Autodesk Fusion 360 part; units mm, degrees
note: some values were not read from the file. Set by a fixed rule: the direction of a hole.
(part 3 of 4)
sketch "草图3" plane through (0, 0, 0) normal (0, 0, 1) x (-1, 0, 0)
  circle A0 centre (-13.5, -30) radius 1.6
  circle A1 centre (0, -30) radius 9
  circle A2 centre (13.5, -30) radius 1.6
  circle A3 centre (6.75, -41.6913) radius 1.6
  circle A4 centre (6.75, -18.3087) radius 1.6
  circle A5 centre (-6.75, -18.3087) radius 1.6
  circle A6 centre (-6.75, -41.6913) radius 1.6
  arc A7 (27.4762, -17.824) -> (28.5, -13.9083) centre (20.5, -13.9083) ccw
  line L0 (28.5, -13.9083) -> (28.5, 0)
  line L1 (28.5, 0) -> (-28.5, 0)
  line L2 (-28.5, 0) -> (-28.5, -13.9083)
  arc A8 (-28.5, -13.9083) -> (-27.4762, -17.824) centre (-20.5, -13.9083) ccw
  line L3 (-27.4762, -17.824) -> (-15.6964, -38.8105)
  arc A9 (-15.6964, -38.8105) -> (15.6964, -38.8105) centre (0, -30) ccw
  line L4 (15.6964, -38.8105) -> (27.4762, -17.824)
  line L5 (0, 0) -> (0, -30) construction
  line L6 (-23.5, -6) -> (-23.5, -14.6927)
  line L7 (-23.5, -14.6927) -> (-18.1186, -24.28)
  line L8 (-23.5, -6) -> (-3, -6)
  line L9 (-3, -6) -> (-3, -11.2383)
  arc A10 (-3, -11.2383) -> (-18.1186, -24.28) centre (0, -30) ccw
  line L10 (-23.5, -6) -> (-28.5, -6) construction
  line L11 (-23.5, -6) -> (-23.5, 0) construction
  line L12 (-18.1186, -24.28) -> (-22.4787, -26.7274) construction
  line L13 (-3, -6) -> (0, -6) construction
  line L14 (23.5, -6) -> (23.5, -14.6927)
  line L15 (23.5, -6) -> (3, -6)
  line L16 (3, -6) -> (3, -11.2383)
  arc A11 (18.1186, -24.28) -> (3, -11.2383) centre (0, -30) ccw
  line L17 (23.5, -14.6927) -> (18.1186, -24.28)
  dimension "d21" = 5
  dimension "d22" = 19
  dimension "d23" = 3
  dimension "d26" = 6
  constraint coincident L5.start origin
  constraint coincident A1.centre A9.centre
  constraint vertical L6
  constraint perpendicular L6 L8
  constraint perpendicular L8 L9
  constraint parallel L3 L7
  constraint coincident L2 L10.end
  constraint perpendicular L2 L10
  constraint coincident L1 L11.end
  constraint perpendicular L1 L11
  constraint coincident L3 L12.end
  constraint perpendicular L3 L12
  constraint coincident L5 L13.end
  constraint perpendicular L5 L13
  constraint symmetric L5 L6.start L14.start
  constraint symmetric L5 L6.end L14.end
  constraint symmetric L5 L8.end L15.end
  constraint symmetric L5 L9.end L16.end
  constraint symmetric L5 L7.end A11.start
  constraint symmetric L5 A10 A11
  constraint equal L10 L12
  measures "d21" distance of L6.start L10.end
  measures "d22" radius of A10
  measures "d23" distance of L8.end L13.end
  measures "d26" distance of L6.start L11.end
extrude "拉伸4" cut sketch "草图3" against normal blind 8 contours L6 L7 L8 L9 A10 | L14 L15 L16 A11 L17
fillet "圆角2" radius 2 8 edges at (18.1186, 24.28, -4) (-18.1186, 24.28, -4) (23.5, 6, -4) (3, 6, -4) (-23.5, 6, -4) (-3, 6, -4) (-3, 11.2383, -4) (3, 11.2383, -4)
fillet "圆角2" radius 6 2 edges at (-23.5, 14.6927, -4) (23.5, 14.6927, -4)
sketch "草图4" plane through (0, 0, 0) normal (0, 0, 1) x (-1, 0, 0)
  arc A0 (27.4762, -17.824) -> (28.5, -13.9083) centre (20.5, -13.9083) ccw
  line L0 (28.5, -13.9083) -> (28.5, 0)
  line L1 (28.5, 0) -> (-28.5, 0)
  line L2 (-28.5, 0) -> (-28.5, -13.9083)
  arc A1 (-28.5, -13.9083) -> (-27.4762, -17.824) centre (-20.5, -13.9083) ccw
  line L3 (-27.4762, -17.824) -> (-15.6964, -38.8105)
  arc A2 (-15.6964, -38.8105) -> (15.6964, -38.8105) centre (0, -30) ccw
  line L4 (15.6964, -38.8105) -> (27.4762, -17.824)
  circle A3 centre (-6.75, -41.6913) radius 1.6
  circle A4 centre (-6.75, -18.3087) radius 1.6
  circle A5 centre (6.75, -18.3087) radius 1.6
  circle A6 centre (6.75, -41.6913) radius 1.6
  circle A7 centre (13.5, -30) radius 1.6
  circle A8 centre (0, -30) radius 9
  circle A9 centre (-13.5, -30) radius 1.6
  line L5 (-20.0922, -20.7639) -> (-22.7321, -16.0607)
  arc A10 (-23.5, -13.1239) -> (-22.7321, -16.0607) centre (-17.5, -13.1239) ccw
  line L6 (-23.5, -13.1239) -> (-23.5, -8)
  arc A11 (-21.5, -6) -> (-23.5, -8) centre (-21.5, -8) ccw
  line L7 (-21.5, -6) -> (-5, -6)
  arc A12 (-3, -8) -> (-5, -6) centre (-5, -8) ccw
  line L8 (-3, -8) -> (-3, -9.6039)
  arc A13 (-4.5238, -11.5464) -> (-3, -9.6039) centre (-5, -9.6039) ccw
  arc A14 (-4.5238, -11.5464) -> (-16.6007, -20.7579) centre (0, -30) ccw
  arc A15 (-20.0922, -20.7639) -> (-16.6007, -20.7579) centre (-18.3481, -19.785) ccw
  line L9 (3, -9.6039) -> (3, -8)
  arc A16 (5, -6) -> (3, -8) centre (5, -8) ccw
  line L10 (5, -6) -> (21.5, -6)
  arc A17 (23.5, -8) -> (21.5, -6) centre (21.5, -8) ccw
  line L11 (23.5, -8) -> (23.5, -13.1239)
  arc A18 (22.7321, -16.0607) -> (23.5, -13.1239) centre (17.5, -13.1239) ccw
  line L12 (22.7321, -16.0607) -> (20.0922, -20.7639)
  arc A19 (16.6007, -20.7579) -> (20.0922, -20.7639) centre (18.3481, -19.785) ccw
  arc A20 (16.6007, -20.7579) -> (4.5238, -11.5464) centre (0, -30) ccw
  arc A21 (3, -9.6039) -> (4.5238, -11.5464) centre (5, -9.6039) ccw
  circle A22 centre (-13.5, -30) radius 3
  circle A23 centre (-6.75, -41.6913) radius 3
  circle A24 centre (6.75, -41.6913) radius 3
  circle A25 centre (13.5, -30) radius 3
  circle A26 centre (6.75, -18.3087) radius 3
  circle A27 centre (-6.75, -18.3087) radius 3
  dimension "d31" = 6
  dimension "d33" = 360
  constraint concentric A9 A22
  measures "d31" diameter of A22
extrude "拉伸5" cut sketch "草图4" against normal blind 3.2 contours A22 | A23 | A24 | A25 | A26 | A27

design "深沟球20，27，4"
part number: 2026-07-22-11-56-50-553
Autodesk Fusion 360 part; units mm, degrees
sketch "草图1" plane through (0, 0, 0) normal (0, 0, 1) x (1, 0, 0)
  circle A0 centre (0, 0) radius 13.5
  circle A1 centre (0, 0) radius 10
  dimension "d1" = 27
  dimension "d2" = 20
  constraint coincident A0.centre A1.centre
  constraint concentric A0 A1
  measures "d1" diameter of A0
  measures "d2" diameter of A1
extrude "拉伸1" add sketch "草图1" along normal blind 3.2
sketch "草图2" plane through (0, 0, 3.2) normal (0, 0, 1) x (1, 0, 0)
  circle A0 centre (0, 0) radius 10
  circle A1 centre (0, 0) radius 13.5
  circle A2 centre (0, 0) radius 14.25
  dimension "d5" = 28.5
  constraint coincident A0.centre A1.centre
  measures "d5" diameter of A2
extrude "拉伸2" add sketch "草图2" along normal blind 0.8 contours A1 | A2

design "yaw输出cnc"
part number: 2026-07-21-18-54-59-892
Autodesk Fusion 360 part; units mm, degrees
sketch "草图1" plane through (0, 0, 0) normal (0, 0, 1) x (1, 0, 0)
  circle A0 centre (0, 0) radius 17.5
  circle A1 centre (0, 0) radius 13.5 construction
  circle A2 centre (-13.5, 0) radius 1.8
  circle A3 centre (-6.75, -11.6913) radius 1.8
  circle A4 centre (6.75, -11.6913) radius 1.8
  circle A5 centre (13.5, 0) radius 1.8
  circle A6 centre (6.75, 11.6913) radius 1.8
  circle A7 centre (-6.75, 11.6913) radius 1.8
  dimension "d1" = 35
  dimension "d2" = 27
  dimension "d3" = 3.6
  dimension "d5" = 360
  constraint coincident A0.centre A1.centre
  constraint concentric A0 A1
  constraint coincident A1 A2.centre
  constraint horizontal A2.centre A5.centre
  measures "d1" diameter of A0
  measures "d2" diameter of A1
  measures "d3" diameter of A2
extrude "拉伸1" add sketch "草图1" along normal blind 7.6
sketch "草图2" plane through (0, 0, 7.6) normal (0, 0, 1) x (-1, 0, 0)
  circle A0 centre (-6.75, 11.6913) radius 1.8
  circle A1 centre (6.75, -11.6913) radius 1.8
  circle A2 centre (13.5, 0) radius 1.8
  circle A3 centre (-13.5, 0) radius 1.8
  circle A4 centre (-6.75, -11.6913) radius 1.8
  circle A5 centre (6.75, 11.6913) radius 1.8
  circle A6 centre (0, 0) radius 17.5
  circle A7 centre (0, 0) radius 19
  dimension "d9" = 38
  constraint concentric A6 A7
  measures "d9" diameter of A7
extrude "拉伸2" add sketch "草图2" along normal blind 6 contours A6 | A7
sketch "草图10" plane through (0, 0, 13.6) normal (0, 0, 1) x (-1, 0, 0)
  circle A0 centre (-6.75, -11.6913) radius 1.8
  circle A1 centre (6.75, -11.6913) radius 1.8
  circle A2 centre (13.5, 0) radius 1.8
  circle A3 centre (-13.5, 0) radius 1.8
  circle A4 centre (-6.75, 11.6913) radius 1.8
  circle A5 centre (6.75, 11.6913) radius 1.8
  circle A6 centre (0, 0) radius 19
  circle A7 centre (0, 0) radius 8
  dimension "d51" = 16
  constraint coincident A6.centre A7.centre
  measures "d51" diameter of A7
extrude "拉伸9" cut sketch "草图10" against normal blind 47 contours A7
sketch "草图11" plane through (0, 0, 13.6) normal (0, 0, 1) x (-1, 0, 0)
  circle A0 centre (0, 0) radius 8
  circle A1 centre (-6.75, -11.6913) radius 1.8
  circle A2 centre (6.75, -11.6913) radius 1.8
  circle A3 centre (13.5, 0) radius 1.8
  circle A4 centre (-13.5, 0) radius 1.8
  circle A5 centre (-6.75, 11.6913) radius 1.8
  circle A6 centre (6.75, 11.6913) radius 1.8
  circle A7 centre (0, 0) radius 19
  line L0 (0, 0) -> (24.6202, -4.3412)
  line L1 (0, 0) -> (24, 0)
  line L2 (0, 0) -> (24.6202, 4.3412)
  circle A8 centre (0, 0) radius 25
  circle A9 centre (0, 0) radius 19
  dimension "d56" = 10
  dimension "d57" = 10
  dimension "d63" = 50
  constraint coincident A0.centre A7.centre
  constraint horizontal L1
  constraint concentric A0 A8
  constraint coincident L0.end A8
  constraint coincident L2.end A8
  measures "d56" angle of L0 L1
  measures "d57" angle of L1 L2
  measures "d63" diameter of A8
extrude "拉伸10" add sketch "草图11" against normal blind 3 contours A7 L0 L2 A8 A9 picked at (22.8867, -2.1872)
fillet "圆角1" radius 1 4 edges at (-18.7113, 3.2993, 12.1) (-24.6202, 4.3412, 12.1) (-24.6202, -4.3412, 12.1) (-18.7113, -3.2993, 12.1)
equation "d38 = ( 45 / 4 ) * 1 mm"
equation "d69 = '7.4'"

design "l2电机固定前"
part number: 2026-07-22-11-09-26-482
Autodesk Fusion 360 part; units mm, degrees
sketch "草图1" plane through (0, 0, 0) normal (0, 0, 1) x (1, 0, 0)
  circle A0 centre (0, 50.1368) radius 25 construction
  circle A1 centre (0, 50.1368) radius 20
  circle A2 centre (0, 50.1368) radius 30
  circle A3 centre (-22.6577, 60.7023) radius 1.6
  circle A4 centre (-20.4788, 35.7974) radius 1.6
  circle A5 centre (2.1789, 25.232) radius 1.6
  circle A6 centre (22.6577, 39.5714) radius 1.6
  circle A7 centre (20.4788, 64.4762) radius 1.6
  circle A8 centre (-2.1789, 75.0417) radius 1.6
  line L0 (-22.5, 10.1368) -> (22.5, 10.1368)
  line L1 (0, 10.1368) -> (0, 50.1368)
  line L2 (6.1726, 76.5877) -> (6.1726, 78.4678)
  circle A9 centre (0, 50.1368) radius 18
  line L3 (0, 50.1368) -> (0, 87.9264)
  line L4 (-29.4017, 44.1753) -> (-22.5, 10.1368)
  line L5 (22.5, 10.1368) -> (29.4017, 44.1753)
  line L6 (-22.6577, 60.7023) -> (0, 50.1368) construction
  dimension "d1" = 50
  dimension "d2" = 40
  dimension "d3" = 60
  dimension "d4" = 3.2
  dimension "d6" = 360
  dimension "d9" = 40
  dimension "d12" = 22.5
  dimension "d79" = 65
  constraint concentric A0 A1
  constraint concentric A1 A2
  constraint horizontal L0
  constraint vertical origin A0.centre
  constraint midpoint L0 L1.start
  constraint coincident A0.centre A1.centre
  constraint coincident A0 A3.centre
  constraint parallel L2 L3
  constraint vertical L1
  constraint coincident A2 L4.start
  constraint coincident A2 L5.end
  constraint tangent A2 L5
  constraint tangent A2 L4
  constraint coincident A3.centre L6.start
  constraint vertical L3
  measures "d1" diameter of A0
  measures "d2" diameter of A1
  measures "d3" diameter of A2
  measures "d4" diameter of A3
  measures "d9" distance of A0.centre L0
  measures "d12" distance of L0.start L1
  measures "d79" angle of L3 L6
extrude "拉伸1" add sketch "草图1" along normal blind 4 contours A1 A2 L1 L3 | A1 A2 L1 L3 | A2 L0 L1 L4 | A2 L0 L1 L5 | A3 | A4 | A5 | A6 | A7 | A8
sketch "草图2" plane through (0, 0, 0) normal (0, 0, -1) x (-1, 0, 0)
  circle A0 centre (-17.5, 13.1368) radius 1.65
  circle A1 centre (0, 13.1368) radius 1.65
  circle A2 centre (17.5, 13.1368) radius 1.65
  line L0 (-29.4017, 44.1753) -> (-22.5, 10.1368)
  line L1 (-22.5, 10.1368) -> (22.5, 10.1368)
  line L2 (22.5, 10.1368) -> (29.4017, 44.1753)
  arc A3 (29.4017, 44.1753) -> (-29.4017, 44.1753) centre (0, 50.1368) ccw
  circle A4 centre (0, 50.1368) radius 20
  dimension "d13" = 3.3
  dimension "d18" = 35
  dimension "d19" = 0
  dimension "d29" = 3
  dimension "d40" = 5
  measures "d13" diameter of A0
  measures "d29" distance of A0.centre L1
  measures "d40" horizontal distance of A0.centre L0.end
extrude "拉伸2" cut sketch "草图2" against normal blind 10 contours A0 | A1 | A2
sketch "草图4" plane through (0, 0, 0) normal (0, 0, -1) x (-1, 0, 0)
  line L0 (-29.4017, 44.1753) -> (-22.5, 10.1368)
  line L1 (-22.5, 10.1368) -> (22.5, 10.1368)
  line L2 (22.5, 10.1368) -> (29.4017, 44.1753)
  arc A0 (29.4017, 44.1753) -> (-29.4017, 44.1753) centre (0, 50.1368) ccw
  circle A1 centre (-17.5, 13.1368) radius 1.65
  circle A2 centre (17.5, 13.1368) radius 1.65
  circle A3 centre (0, 13.1368) radius 1.65
  circle A4 centre (-17.5, 13.1368) radius 3
  line L3 (-20.5, 13.1368) -> (-20.5, 10.1368)
  line L4 (-14.5, 13.1368) -> (-14.5, 10.1368)
  circle A5 centre (0, 13.1368) radius 3
  line L5 (3, 13.1368) -> (3, 10.1368)
  line L6 (-3, 13.1368) -> (-3, 10.1368)
  circle A6 centre (17.5, 13.1368) radius 3
  line L7 (20.5, 13.1368) -> (20.5, 10.1368)
  line L8 (14.5, 13.1368) -> (14.5, 10.1368)
  circle A7 centre (0, 50.1368) radius 20
  dimension "d36" = 35
  dimension "d37" = 0
  constraint concentric A1 A4
  constraint tangent L1 A4
  constraint coincident A4 L3.start
  constraint coincident L1 L3.end
  constraint tangent A4 L3
  constraint vertical L3
  constraint coincident A4 L4.start
  constraint coincident L1 L4.end
  constraint perpendicular L1 L4
  constraint tangent A4 L4
hole "孔1" at (2.1789, 25.232, 0) at (-20.4788, 35.7974, 0) at (-22.6577, 60.7023, 0) at (-2.1789, 75.0417, 0) at (20.4788, 64.4762, 0) at (22.6577, 39.5714, 0) direction (0, 0, 1) diameter 3.3 depth 7 tip angle 180 countersink diameter 6.3 countersink angle 90
sketch "草图5" plane through (0, 0, 0) normal (0, 0, 1) x (1, 0, 0)
  circle A0 centre (17.5, 13.1368) radius 1.65
  circle A1 centre (0, 13.1368) radius 1.65
  circle A2 centre (-17.5, 13.1368) radius 1.65
  circle A3 centre (0, 50.1368) radius 20
  line L0 (22.5, 10.1368) -> (29.4017, 44.1753)
  arc A4 (29.4017, 44.1753) -> (-29.4017, 44.1753) centre (0, 50.1368) ccw
  line L1 (-29.4017, 44.1753) -> (-22.5, 10.1368)
  line L2 (-22.5, 10.1368) -> (22.5, 10.1368)
  circle A5 centre (-25, 50.1368) radius 1.6
  circle A6 centre (12.5, 28.4862) radius 1.6
  circle A7 centre (12.5, 71.7875) radius 1.6
  circle A8 centre (-12.5, 71.7875) radius 1.6
  circle A9 centre (25, 50.1368) radius 1.6
  circle A10 centre (-12.5, 28.4862) radius 1.6
  circle A11 centre (0, 50.1368) radius 25
  line L3 (75, 70.1368) -> (-75, 70.1368)
  arc A12 (-75, 70.1368) -> (-75, 30.1368) centre (-75, 50.1368) ccw
  line L4 (-75, 30.1368) -> (75, 30.1368)
  arc A13 (75, 30.1368) -> (75, 70.1368) centre (75, 50.1368) ccw
  line L5 (75, 50.1368) -> (-75, 50.1368) construction
  line L6 (-40, 30.1368) -> (-3.2298, 25.3463)
  circle A14 centre (17.5, 13.1368) radius 1.65
  circle A15 centre (0, 13.1368) radius 1.65
  circle A16 centre (-17.5, 13.1368) radius 1.65
  circle A17 centre (0, 50.1368) radius 20
  line L7 (29.4017, 44.1753) -> (22.5, 10.1368)
  line L8 (22.5, 10.1368) -> (-22.5, 10.1368)
  line L9 (-22.5, 10.1368) -> (-29.4017, 44.1753)
  arc A18 (29.4017, 44.1753) -> (-29.4017, 44.1753) centre (0, 50.1368) ccw
  circle A19 centre (2.1789, 25.232) radius 3.15
  circle A20 centre (0, 50.1368) radius 30
  line L10 (3.2298, 25.3463) -> (40, 30.1368)
  circle A21 centre (22.6577, 39.5714) radius 3.15
  circle A22 centre (-2.1789, 75.0417) radius 3.15
  circle A23 centre (-20.4788, 35.7974) radius 3.15
  circle A24 centre (-22.6577, 60.7023) radius 3.15
  circle A25 centre (20.4788, 64.4762) radius 3.15
  line L11 (24.0557, 17.8092) -> (-24.0557, 17.8092)
  line L12 (24.0557, 17.8092) -> (-6.4705, 25.9887)
  point P0 (0, 50.1368)
  dimension "d46" = 50
  dimension "d47" = 20
  dimension "d48" = 40
  dimension "d75" = 60
  dimension "d76" = 40
  dimension "d84" = 15
  constraint concentric A3 A11
  constraint tangent L3 A12
  constraint tangent A12 L4
  constraint parallel L3 L4
  constraint tangent L4 A13
  constraint tangent L3 A13
  constraint horizontal L5
  constraint coincident P0 A3.centre
  constraint midpoint L5 P0
  constraint coincident L4 L6.start
  constraint coincident A11 L6.end
  constraint tangent A11 L6
  constraint concentric A17 A20
  constraint coincident A11 L10.start
  constraint coincident L4 L10.end
  constraint tangent A11 L10
  constraint coincident L7 L11.start
  constraint coincident L9 L11.end
  constraint horizontal L11
  constraint coincident A11 L12.end
  constraint tangent A11 L12
  measures "d46" diameter of A11
  measures "d47" radius of A12
  measures "d48" horizontal distance of P0 L6.start
  measures "d75" diameter of A20
  measures "d76" horizontal distance of P0 L10.end
  measures "d84" angle of L11 L12
extrude "拉伸5" add sketch "草图5" against normal blind 6 contours L1 L6 L9 A20 L11 L12 | L0 L1 L2 L7 L8 L9 L11
fillet "圆角1" radius 2 7 edges at (-22.5, 10.1368, -1) (22.5, 10.1368, 2) (22.5, 10.1368, -3) (24.0557, 17.8092, -3) (9.5476, 21.6966, -3) (-19.6739, 27.4887, -3) (-26.1904, 28.3377, -3)
sketch "草图6" plane through (0, 0, -6) normal (0, 0, -1) x (1, 0, 0)
  line L0 (-22.8249, -11.7394) -> (-25.6344, -25.5955)
  line L1 (20.8648, -10.1368) -> (-20.8648, -10.1368)
  line L2 (23.682, -15.9666) -> (22.8249, -11.7394)
  line L3 (0, 0) -> (0, -50.1368)
  line L4 (-21.7001, -21.2885) -> (-5, -17.1368)
  line L5 (-5, -17.1368) -> (-19.3031, -17.1368)
  line L6 (-19.3031, -17.1368) -> (-21.7001, -21.2885)
  line L7 (5, -17.1368) -> (19.3031, -17.1368)
  line L8 (19.3031, -17.1368) -> (21.7001, -21.2885)
  line L9 (21.7001, -21.2885) -> (5, -17.1368)
  arc A0 (9.0021, -21.5193) -> (-19.2373, -27.1167) centre (0, -50.1368) ccw
  circle A1 centre (17.5, -13.1368) radius 1.65
  circle A2 centre (0, -13.1368) radius 1.65
  circle A3 centre (-17.5, -13.1368) radius 1.65
  arc A4 (22.8249, -11.7394) -> (20.8648, -10.1368) centre (20.8648, -12.1368) ccw
  arc A5 (-20.8648, -10.1368) -> (-22.8249, -11.7394) centre (-20.8648, -12.1368) ccw
  line L10 (-23.4159, -27.9762) -> (-20.2614, -27.5652)
  line L11 (10.1198, -21.5433) -> (22.2396, -18.2958)
  arc A6 (-25.6344, -25.5955) -> (-23.4159, -27.9762) centre (-23.6743, -25.993) ccw
  arc A7 (-20.2614, -27.5652) -> (-19.2373, -27.1167) centre (-20.5198, -25.582) ccw
  arc A8 (9.0021, -21.5193) -> (10.1198, -21.5433) centre (9.6022, -19.6115) ccw
  arc A9 (22.2396, -18.2958) -> (23.682, -15.9666) centre (21.7219, -16.364) ccw
  dimension "d69" = 5
  dimension "d71" = 120
  constraint coincident L3.start origin
  constraint horizontal L5
  constraint symmetric L3 L4.start L8.end
  constraint symmetric L3 L4.end L7.start
  constraint symmetric L3 L5.end L7.end
  measures "d69" distance of L3 L4.end
  measures "d71" angle of L5 L6
sketch "草图7" plane through (0, 0, -6) normal (0, 0, -1) x (1, 0, 0)
  line L0 (-22.8249, -11.7394) -> (-25.6344, -25.5955)
  line L1 (23.682, -15.9666) -> (22.8249, -11.7394)
  circle A0 centre (-17.5, -13.1368) radius 3
  line L2 (-20.5, -13.1368) -> (-20.5, -10.1368)
  line L3 (-14.5, -13.1368) -> (-14.5, -10.0707)
  line L4 (20.8648, -10.1368) -> (-20.8648, -10.1368)
  arc A1 (9.0021, -21.5193) -> (-19.2373, -27.1167) centre (0, -50.1368) ccw
  circle A2 centre (17.5, -13.1368) radius 1.65
  circle A3 centre (0, -13.1368) radius 1.65
  circle A4 centre (-17.5, -13.1368) radius 1.65
  arc A5 (22.8249, -11.7394) -> (20.8648, -10.1368) centre (20.8648, -12.1368) ccw
  arc A6 (-20.8648, -10.1368) -> (-22.8249, -11.7394) centre (-20.8648, -12.1368) ccw
  line L5 (-23.4159, -27.9762) -> (-20.2614, -27.5652)
  line L6 (10.1198, -21.5433) -> (22.2396, -18.2958)
  arc A7 (-25.6344, -25.5955) -> (-23.4159, -27.9762) centre (-23.6743, -25.993) ccw
  arc A8 (-20.2614, -27.5652) -> (-19.2373, -27.1167) centre (-20.5198, -25.582) ccw
  arc A9 (9.0021, -21.5193) -> (10.1198, -21.5433) centre (9.6022, -19.6115) ccw
  arc A10 (22.2396, -18.2958) -> (23.682, -15.9666) centre (21.7219, -16.364) ccw
  dimension "d62" = 6
  constraint coincident A0 L2.start
  constraint coincident A0 L3.start
  constraint vertical L3
  constraint vertical L2
  constraint tangent A0 L3
  constraint tangent A0 L2
  constraint coincident L2.end L4
  measures "d62" diameter of A0
extrude "拉伸7" cut sketch "草图7" against normal blind 3 contours A0 L2 L4 | A0 | A0 L3 L4 | A4
pattern_linear "R-阵列2" count 3 spacing 17.5 along (1, 0, 0) of "拉伸7"

design "M3铝柱 55mm"
part number: 2026-08-11-12-14-30-494
Autodesk Fusion 360 part; units mm, degrees
sketch "草图1" plane through (0, 0, 0) normal (0, 1, 0) x (1, 0, 0)
  circle A0 centre (0, 0) radius 1.5
  circle A1 centre (0, 0) radius 3
  dimension "d1" = 3
  dimension "d2" = 6
  constraint coincident A0.centre A1.centre
  measures "d1" diameter of A0
  measures "d2" diameter of A1
extrude "拉伸1" add sketch "草图1" along normal mid plane 55 makes body 1
pattern_linear "R-阵列1" count 2 spacing 50 along (1, 0, 0) count 2 spacing 30 along (0, 0, 1) of bodies 1 makes body 2 at (52.9851, 9.1667, 0.2987) makes body 3 at (2.9851, 9.1667, 30.2987) makes body 4 at (52.9851, 9.1667, 30.2987)

design "深沟球35*44*5"
part number: 2026-07-21-18-41-33-064
Autodesk Fusion 360 part; units mm, degrees
sketch "草图1" plane through (0, 0, 0) normal (0, 0, 1) x (1, 0, 0)
  circle A0 centre (0, 0) radius 17.5
  circle A1 centre (0, 0) radius 22
  dimension "d1" = 35
  dimension "d2" = 44
  constraint coincident A0.centre A1.centre
  measures "d1" diameter of A0
  measures "d2" diameter of A1
extrude "拉伸1" add sketch "草图1" along normal blind 5

design "滑块底座"
part number: 2026-07-22-10-29-59-170
Autodesk Fusion 360 part; units mm, degrees
sketch "草图1" plane through (0, 0, 0) normal (0, 1, 0) x (1, 0, 0)
  line L0 (0, 0) -> (0, -4.5) construction
  line L1 (0, 0) -> (-20, 0)
  line L2 (-20, 0) -> (-20, -7)
  line L3 (-20, -7) -> (-8.6, -7)
  line L4 (-8.6, -7) -> (-8.6, -4.5)
  line L5 (-8.6, -4.5) -> (0, -4.5)
  line L6 (20, 0) -> (20, -7)
  line L7 (20, -7) -> (8.6, -7)
  line L8 (8.6, -7) -> (8.6, -4.5)
  line L9 (8.6, -4.5) -> (0, -4.5)
  line L10 (0, 0) -> (20, 0)
  dimension "d1" = 40
  dimension "d2" = 7
  dimension "d4" = 2.5
  dimension "d16" = 17.2
  constraint coincident L0.start L1.start
  constraint vertical L0
  constraint perpendicular L0 L1
  constraint perpendicular L1 L2
  constraint perpendicular L2 L3
  constraint perpendicular L3 L4
  constraint perpendicular L0 L5
  constraint symmetric L1.start L0 L10.start
  constraint symmetric L5.end L0 L9.end
  constraint symmetric L0 L3.end L7.end
  constraint symmetric L0 L4.end L8.end
  constraint symmetric L0 L2.end L6.end
  constraint horizontal L10
  measures "d1" distance of L2 L6
  measures "d2" distance of L1.end L2.end
  measures "d4" distance of L3.end L4.end
  measures "d16" distance of L4 L8
extrude "拉伸1" add sketch "草图1" along normal mid plane 22.5
sketch "草图2" plane through (0, 0, 0) normal (0, 0, 1) x (-1, 0, 0)
  line L0 (-8.6, 11.25) -> (-8.6, -11.25)
  line L1 (-8.6, -11.25) -> (8.6, -11.25)
  line L2 (8.6, -11.25) -> (8.6, 11.25)
  line L3 (8.6, 11.25) -> (-8.6, 11.25)
  line L4 (0, -11.25) -> (0, 11.25) construction
  line L5 (8.6, 0) -> (-8.6, 0) construction
  circle A0 centre (6, -4) radius 1.75
  circle A1 centre (-6, -4) radius 1.75
  circle A2 centre (6, 4) radius 1.75
  circle A3 centre (-6, 4) radius 1.75
  line L6 (20, 11.25) -> (20, -11.25)
  line L7 (20, -11.25) -> (-20, -11.25)
  line L8 (-20, -11.25) -> (-20, 11.25)
  line L9 (-20, 11.25) -> (20, 11.25)
  dimension "d7" = 3.5
  dimension "d8" = 8
  dimension "d9" = 12
  constraint midpoint L1 L4.start
  constraint perpendicular L1 L4
  constraint midpoint L2 L5.start
  constraint midpoint L0 L5.end
  constraint equal A0 A1
  constraint equal A1 A3
  constraint equal A2 A3
  constraint symmetric L4 A0.centre A1.centre
  constraint symmetric L5 A1.centre A3.centre
  constraint symmetric L4 A2.centre A3.centre
  constraint midpoint L3 L4.end
  measures "d7" diameter of A0
  measures "d8" distance of A0.centre A2.centre
  measures "d9" distance of A0.centre A1.centre
hole "孔2" at (6, -4, 0) at (6, 4, 0) at (-6, -4, 0) at (-6, 4, 0) direction (0, 0, 1) diameter 2.2 depth 6 tip angle 180 counterbore diameter 4 counterbore depth 2.5
sketch "草图5" plane through (0, 0, 7) normal (0, 0, 1) x (-1, 0, 0)
  line L0 (8.6, 11.25) -> (8.6, -11.25)
  line L1 (8.6, -11.25) -> (20, -11.25)
  line L2 (20, -11.25) -> (20, 11.25)
  line L3 (20, 11.25) -> (8.6, 11.25)
  line L4 (20, 0) -> (8.6, 0) construction
  circle A0 centre (16, 0) radius 1.25
  dimension "d20" = 2.5
  dimension "d23" = 16
  constraint midpoint L2 L4.start
  constraint midpoint L0 L4.end
  constraint coincident L4 A0.centre
  measures "d20" diameter of A0
  measures "d23" distance of origin A0.centre
extrude "拉伸4" cut sketch "草图5" against normal up to surface (7 mm away) contours A0
sketch "草图6" plane through (0, 0, 7) normal (0, 0, 1) x (-1, 0, 0)
  circle A0 centre (16, 0) radius 1.25
  line L0 (8.6, 11.25) -> (8.6, -11.25)
  line L1 (8.6, -11.25) -> (20, -11.25)
  line L2 (20, -11.25) -> (20, 11.25)
  line L3 (20, 11.25) -> (8.6, 11.25)
  circle A1 centre (16, 0) radius 1.25
  circle A2 centre (16, 0) radius 2.5
  dimension "d24" = 2.5
  dimension "d25" = 5
  constraint concentric A0 A1
  constraint concentric A1 A2
  measures "d24" diameter of A1
  measures "d25" diameter of A2
extrude "拉伸5" add sketch "草图6" along normal blind 1 contours A2
sketch "草图7" plane through (0, 0, 7) normal (0, 0, 1) x (-1, 0, 0)
  line L0 (-20, 11.25) -> (-20, -11.25)
  line L1 (-20, -11.25) -> (-8.6, -11.25)
  line L2 (-8.6, -11.25) -> (-8.6, 11.25)
  line L3 (-8.6, 11.25) -> (-20, 11.25)
  line L4 (-20, -11.25) -> (-11, -11.25)
  line L5 (-11, -11.25) -> (-11, 11.25)
  line L6 (-11, 11.25) -> (-20, 11.25)
  line L7 (-20, 11.25) -> (-20, -11.25)
  dimension "d28" = 9
  constraint horizontal L4
  constraint vertical L5
  constraint horizontal L6
  constraint vertical L7
  constraint coincident L3 L5.end
  constraint coincident L0.end L1.start
  measures "d28" distance of L0.end L4.end
extrude "拉伸6" cut sketch "草图7" against normal blind 3.5 contours L0 L1 L3 L4 L5 L6 L7
sketch "草图9" plane through (0, 0, 0) normal (0, 0, -1) x (1, 0, 0)
  circle A0 centre (-16, 0) radius 1.25
  line L0 (-20, 11.25) -> (-20, -11.25)
  line L1 (-20, -11.25) -> (20, -11.25)
  line L2 (20, -11.25) -> (20, 11.25)
  line L3 (20, 11.25) -> (-20, 11.25)
  line L4 (0, 11.25) -> (0, -11.25) construction
  line L5 (-20, 0) -> (20, 0) construction
  circle A1 centre (-16, 8) radius 1.5
  circle A2 centre (-16, -8) radius 1.5
  circle A3 centre (16, 8) radius 1.5
  circle A4 centre (16, -8) radius 1.5
  circle A5 centre (-6, 4) radius 2
  circle A6 centre (6, 4) radius 2
  circle A7 centre (6, -4) radius 2
  circle A8 centre (-6, -4) radius 2
  dimension "d31" = 3
  dimension "d32" = 16
  dimension "d33" = 32
  constraint midpoint L3 L4.start
  constraint perpendicular L3 L4
  constraint midpoint L0 L5.start
  constraint midpoint L2 L5.end
  constraint equal A1 A3
  constraint equal A3 A4
  constraint equal A2 A4
  constraint symmetric L4 A1.centre A3.centre
  constraint symmetric L5 A3.centre A4.centre
  constraint symmetric L4 A2.centre A4.centre
  constraint midpoint L1 L4.end
  measures "d31" diameter of A1
  measures "d32" distance of A1.centre A2.centre
  measures "d33" distance of A1.centre A3.centre
hole "孔1" at (-16, -8, 0) at (-16, 8, 0) at (16, -8, 0) at (16, 8, 0) direction (0, 0, 1) diameter 2.5 depth 8 tip angle 180
sketch "草图10" plane through (0, 0, 0) normal (0, 0, -1) x (1, 0, 0)
  line L0 (-20, 11.25) -> (-20, -11.25)
  line L1 (-20, -11.25) -> (20, -11.25)
  line L2 (20, -11.25) -> (20, 11.25)
  line L3 (20, 11.25) -> (-20, 11.25)
  circle A0 centre (-6, -4) radius 2
  circle A1 centre (6, -4) radius 2
  circle A2 centre (6, 4) radius 2
  circle A3 centre (-6, 4) radius 2
  circle A4 centre (-16, 0) radius 1.25
  circle A5 centre (16, -8) radius 1.25
  circle A6 centre (-16, -8) radius 1.25
  circle A7 centre (-16, 8) radius 1.25
  circle A8 centre (16, 8) radius 1.25
hole "孔3" at (0, 0, 0) direction (0, 0, 1) diameter 2.5 depth 6 tip angle 180
fillet "圆角1" radius 3 4 edges at (20, 11.25, 1.75) (20, -11.25, 1.75) (-20, 11.25, 3.5) (-20, -11.25, 3.5)

design "J6轴头_2"
part number: 2026-07-23-15-12-30-457
Autodesk Fusion 360 part; units mm, degrees
sketch "草图1" plane through (0, 0, 0) normal (0, 0, 1) x (1, 0, 0)
  circle A0 centre (0, 0) radius 28.5
  circle A1 centre (0, 0) radius 13.5 construction
  line L0 (0, 0) -> (0, 28.5) construction
  circle A2 centre (0, 13.5) radius 1.6
  circle A3 centre (-11.6913, 6.75) radius 1.6
  circle A4 centre (-11.6913, -6.75) radius 1.6
  circle A5 centre (0, -13.5) radius 1.6
  circle A6 centre (11.6913, -6.75) radius 1.6
  circle A7 centre (11.6913, 6.75) radius 1.6
  circle A8 centre (0, 0) radius 32.5 construction
  circle A9 centre (0, 0) radius 28.5 construction
  circle A10 centre (0, 0) radius 17.5
  circle A11 centre (0, 0) radius 6
  circle A12 centre (22.981, 22.981) radius 1.25
  line L1 (9.1803, 26.981) -> (22.981, 26.981)
  arc A13 (26.981, 22.981) -> (22.981, 26.981) centre (22.981, 22.981) ccw
  line L2 (26.981, 22.981) -> (26.981, 9.1803)
  line L3 (-26.981, 9.1803) -> (-26.981, 22.981)
  arc A14 (-22.981, 26.981) -> (-26.981, 22.981) centre (-22.981, 22.981) ccw
  line L4 (-22.981, 26.981) -> (-9.1803, 26.981)
  circle A15 centre (-22.981, 22.981) radius 1.25
  line L5 (-9.1803, -26.981) -> (-22.981, -26.981)
  arc A16 (-26.981, -22.981) -> (-22.981, -26.981) centre (-22.981, -22.981) ccw
  line L6 (-26.981, -22.981) -> (-26.981, -9.1803)
  circle A17 centre (-22.981, -22.981) radius 1.25
  line L7 (26.981, -9.1803) -> (26.981, -22.981)
  arc A18 (22.981, -26.981) -> (26.981, -22.981) centre (22.981, -22.981) ccw
  line L8 (22.981, -26.981) -> (9.1803, -26.981)
  circle A19 centre (22.981, -22.981) radius 1.25
  dimension "d1" = 57
  dimension "d2" = 27
  dimension "d4" = 360
  dimension "d5" = 3.2
  dimension "d46" = 57
  dimension "d48" = 65
  dimension "d51" = 35
  dimension "d59" = 12
  dimension "d86" = 2.5
  dimension "d87" = 4
  dimension "d89" = 360
  constraint coincident A0.centre A1.centre
  constraint concentric A0 A1
  constraint coincident A0 L0.end
  constraint vertical L0
  constraint coincident L0 A2.centre
  constraint coincident A1 A2.centre
  constraint concentric A8 A9
  constraint concentric A0 A10
  constraint concentric A10 A11
  constraint coincident A8 A12.centre
  constraint coincident A9 L1.start
  constraint horizontal L1
  constraint tangent L1 A13
  constraint coincident A0 L2.end
  constraint vertical L2
  constraint tangent A13 L2
  constraint coincident A12.centre A13.centre
  constraint symmetric L0 A12.centre A14.centre
  measures "d1" diameter of A0
  measures "d2" diameter of A1
  measures "d5" diameter of A2
  measures "d46" diameter of A9
  measures "d48" diameter of A8
  measures "d51" diameter of A10
  measures "d59" diameter of A11
  measures "d86" diameter of A12
  measures "d87" radius of A13
extrude "拉伸1" add sketch "草图1" along normal blind 5 contours A0 | A0 L1 A13 L2 | A0 L7 A18 L8 | A0 L3 A14 L4 | A0 L5 A16 L6 | A10 makes body 1
sketch "草图9" plane through (0, 0, 5) normal (0, 0, 1) x (-1, 0, 0)
  circle A0 centre (-11.6913, -6.75) radius 1.6
  circle A1 centre (0, -13.5) radius 1.6
  circle A2 centre (-11.6913, 6.75) radius 1.6
  circle A3 centre (0, 13.5) radius 1.6
  circle A4 centre (11.6913, -6.75) radius 1.6
  circle A5 centre (11.6913, 6.75) radius 1.6
  circle A6 centre (0, -13.5) radius 3
  circle A7 centre (11.6913, -6.75) radius 3
  circle A8 centre (11.6913, 6.75) radius 3
  circle A9 centre (0, 13.5) radius 3
  circle A10 centre (-11.6913, 6.75) radius 3
  circle A11 centre (-11.6913, -6.75) radius 3
  circle A12 centre (0, 0) radius 6
  circle A13 centre (22.981, 22.981) radius 1.25
  circle A14 centre (22.981, -22.981) radius 1.25
  circle A15 centre (-22.981, 22.981) radius 1.25
  arc A16 (-26.981, 9.1803) -> (-26.981, -9.1803) centre (0, 0) ccw
  line L0 (-26.981, -9.1803) -> (-26.981, -22.981)
  arc A17 (-26.981, -22.981) -> (-22.981, -26.981) centre (-22.981, -22.981) ccw
  line L1 (-22.981, -26.981) -> (-9.1803, -26.981)
  arc A18 (-9.1803, -26.981) -> (9.1803, -26.981) centre (0, 0) ccw
  line L2 (9.1803, -26.981) -> (22.981, -26.981)
  arc A19 (22.981, -26.981) -> (26.981, -22.981) centre (22.981, -22.981) ccw
  line L3 (26.981, -22.981) -> (26.981, -9.1803)
  arc A20 (26.981, -9.1803) -> (26.981, 9.1803) centre (0, 0) ccw
  line L4 (26.981, 9.1803) -> (26.981, 22.981)
  arc A21 (26.981, 22.981) -> (22.981, 26.981) centre (22.981, 22.981) ccw
  line L5 (22.981, 26.981) -> (9.1803, 26.981)
  arc A22 (9.1803, 26.981) -> (-9.1803, 26.981) centre (0, 0) ccw
  line L6 (-9.1803, 26.981) -> (-22.981, 26.981)
  arc A23 (-22.981, 26.981) -> (-26.981, 22.981) centre (-22.981, 22.981) ccw
  line L7 (-26.981, 22.981) -> (-26.981, 9.1803)
  circle A24 centre (-22.981, -22.981) radius 1.25
  dimension "d54" = 6
  dimension "d56" = 360
  constraint concentric A1 A6
  measures "d54" diameter of A6
extrude "拉伸10" cut sketch "草图9" against normal blind 3.2 contours A6 | A7 | A8 | A9 | A10 | A11 bodies 1
sketch "草图11" plane through (0, 0, 0) normal (0, 0, -1) x (1, 0, 0)
  circle A0 centre (-11.6913, 6.75) radius 1.6
  circle A1 centre (-11.6913, -6.75) radius 1.6
  circle A2 centre (11.6913, 6.75) radius 1.6
  circle A3 centre (0, -13.5) radius 1.6
  circle A4 centre (0, 13.5) radius 1.6
  circle A5 centre (0, 0) radius 6
  circle A6 centre (11.6913, -6.75) radius 1.6
  circle A7 centre (0, 0) radius 17.5
  circle A8 centre (0, 0) radius 26
  line L0 (0, 0) -> (0, 26) construction
  line L1 (3.7877, 17.0852) -> (5.6274, 25.3837)
  line L2 (-3.7877, 17.0852) -> (-5.6274, 25.3837)
  dimension "d68" = 35
  dimension "d69" = 52
  dimension "d90" = 25
  constraint concentric A5 A7
  constraint concentric A7 A8
  constraint coincident A5.centre A7.centre
  constraint coincident A8 L0.end
  constraint coincident A7 L1.start
  constraint coincident A8 L1.end
  constraint coincident A5.centre L1
  constraint coincident A7 L2.start
  constraint coincident A8 L2.end
  constraint coincident A5.centre L2
  constraint symmetric L0 L1.start L2.start
  constraint vertical L0
  measures "d68" diameter of A7
  measures "d69" diameter of A8
  measures "d90" angle of L1 L2
extrude "拉伸12" add sketch "草图11" along normal blind 3.5 separate body contours A7 | A7 A8 L1 L2 picked at (-2.9294, 22.9229) makes body 2
extrude "拉伸13" add sketch "草图11" along normal blind 5.5 from surface at 3.5 contours A7 bodies 2
fillet "圆角4" radius 1 2 edges at (5.6274, -25.3837, -1.75) (-5.6274, -25.3837, -1.75) on bodies 2
equation "d69 = ( 26 * 2 ) * 1 mm"

design "滑轨底座"
part number: 2026-07-28-10-26-46-951
Autodesk Fusion 360 part; units mm, degrees
sketch "草图1" plane through (0, 0, 0) normal (0, 0, 1) x (1, 0, 0)
  circle A0 centre (0, 0) radius 20
  circle A1 centre (0, 0) radius 25 construction
  circle A2 centre (0, 0) radius 28.5
  circle A3 centre (-25, 0) radius 1.6
  circle A4 centre (-12.5, -21.6506) radius 1.6
  circle A5 centre (12.5, -21.6506) radius 1.6
  circle A6 centre (25, 0) radius 1.6
  circle A7 centre (12.5, 21.6506) radius 1.6
  circle A8 centre (-12.5, 21.6506) radius 1.6
  line L0 (-28.058, 5) -> (-80, 5)
  line L1 (-80, 5) -> (-80, -5)
  line L2 (-80, -5) -> (-28.058, -5)
  line L3 (0, 0) -> (0, 28.5) construction
  line L4 (0, 0) -> (-80, 0) construction
  circle A9 centre (-75, 0) radius 0.8
  circle A10 centre (-60, 0) radius 0.8
  line L5 (28.058, 5) -> (80, 5)
  line L6 (80, 5) -> (80, -5)
  line L7 (80, -5) -> (28.058, -5)
  circle A11 centre (75, 0) radius 0.8
  circle A12 centre (60, 0) radius 0.8
  circle A13 centre (45, 0) radius 0.8
  circle A14 centre (-45, 0) radius 0.8
  circle A15 centre (-30, 0) radius 0.8
  circle A16 centre (30, 0) radius 0.8
  dimension "d1" = 50
  dimension "d2" = 57
  dimension "d3" = 40
  dimension "d4" = 3.2
  dimension "d6" = 360
  dimension "d7" = 1.6
  dimension "d8" = 10
  dimension "d9" = 160
  dimension "d10" = 5
  dimension "d11" = 15
  dimension "d37" = 15
  dimension "d46" = 15
  constraint coincident A0.centre A1.centre
  constraint concentric A1 A2
  constraint coincident A1 A3.centre
  constraint horizontal A0.centre A3.centre
  constraint coincident A2 L0.start
  constraint horizontal L0
  constraint perpendicular L0 L1
  constraint coincident A2 L2.end
  constraint perpendicular L1 L2
  constraint coincident A2 L3.end
  constraint perpendicular L2 L3
  constraint midpoint L1 L4.end
  constraint horizontal L4
  constraint coincident L4 A9.centre
  constraint coincident L4 A10.centre
  constraint equal A9 A10
  constraint symmetric L0.start L3 L5.start
  constraint symmetric L0.end L3 L5.end
  constraint symmetric L1.end L3 L6.end
  constraint symmetric L2.end L3 L7.end
  constraint symmetric L3 A9 A11
  constraint symmetric L3 A10 A12
  constraint equal A12 A13
  constraint symmetric L3 A13 A14
  constraint coincident L4 A14.centre
  constraint coincident L4 A15.centre
  constraint symmetric L3 A15 A16
  constraint equal A14 A15
  measures "d1" diameter of A1
  measures "d2" diameter of A2
  measures "d3" diameter of A0
  measures "d4" diameter of A3
  measures "d7" diameter of A9
  measures "d8" distance of L0.end L1.end
  measures "d9" distance of L1 L6
  measures "d10" distance of L1 A9.centre
  measures "d11" distance of A9.centre A10.centre
  measures "d37" distance of A10.centre A14.centre
  measures "d46" distance of A14.centre A15.centre
extrude "拉伸1" add sketch "草图1" along normal blind 4 contours A2 | A2 L5 L6 L7 | A2 L0 L1 L2 | A9 | A10 | A11 | A12 | A13 | A14 | A15 | A16
extrude "拉伸2" add sketch "草图1" along normal blind 15 contours A2 L5 L6 L7 | A2 L0 L1 L2 | A9 | A10 | A11 | A12 | A13 | A14 | A15 | A16
fillet "圆角1" radius 12 4 edges at (-28.058, -5, 2) (28.058, -5, 2) (28.058, 5, 2) (-28.058, 5, 2)
sketch "草图2" plane through (0, 0, 15) normal (0, 0, 1) x (-1, 0, 0)
  circle A0 centre (0, 0) radius 28.5
  line L0 (0, 0) -> (0, 28.5) construction
  line L1 (0, 0) -> (-80, 0) construction
  line L2 (-28.2843, 3.5) -> (-80, 3.5)
  line L3 (-80, 3.5) -> (-80, -3.5)
  line L4 (-80, -3.5) -> (-28.2843, -3.5)
  line L5 (80, -3.5) -> (28.2843, -3.5)
  line L6 (80, 3.5) -> (80, -3.5)
  line L7 (28.2843, 3.5) -> (80, 3.5)
  line L8 (-80, -5) -> (-28.058, -5)
  line L9 (-80, 5) -> (-80, -5)
  line L10 (-28.058, 5) -> (-80, 5)
  line L11 (28.058, -5) -> (80, -5)
  line L12 (80, 5) -> (28.058, 5)
  line L13 (80, -5) -> (80, 5)
  dimension "d18" = 160
  dimension "d19" = 57
  dimension "d20" = 7
  constraint coincident A0.centre L0.start
  constraint coincident A0 L0.end
  constraint vertical L0
  constraint perpendicular L0 L1
  constraint coincident A0 L2.start
  constraint horizontal L2
  constraint perpendicular L2 L3
  constraint coincident A0 L4.end
  constraint perpendicular L3 L4
  constraint midpoint L1.end L3
  constraint symmetric L0 L2.start L7.start
  constraint symmetric L0 L2.end L6.start
  constraint symmetric L0 L3.end L5.start
  constraint symmetric L0 L4.end L5.end
  measures "d18" distance of L3 L6
  measures "d19" diameter of A0
  measures "d20" distance of L2.end L3.end
extrude "拉伸3" cut sketch "草图2" against normal blind 11 contours A0 | A0 L7 L12 L13 | A0 L5 L11 L13 | A0 L2 L9 L10 | A0 L4 L8 L9
sketch "草图3" plane through (0, 0, 4) normal (0, 0, 1) x (-1, 0, 0)
  circle A0 centre (25, 0) radius 1.6
  circle A1 centre (-12.5, 21.6506) radius 1.6
  circle A2 centre (-12.5, -21.6506) radius 1.6
  circle A3 centre (-25, 0) radius 1.6
  circle A4 centre (0, 0) radius 20
  circle A5 centre (12.5, 21.6506) radius 1.6
  circle A6 centre (12.5, -21.6506) radius 1.6
  arc A7 (36.7594, -5) -> (25.8677, -11.963) centre (36.7594, -17) ccw
  line L0 (36.7594, -5) -> (80, -5)
  line L1 (80, -5) -> (80, -3.5)
  line L2 (80, -3.5) -> (28.2843, -3.5)
  arc A8 (28.2843, -3.5) -> (28.2843, 3.5) centre (0, 0) ccw
  line L3 (28.2843, 3.5) -> (80, 3.5)
  line L4 (80, 3.5) -> (80, 5)
  line L5 (80, 5) -> (36.7594, 5)
  arc A9 (25.8677, 11.963) -> (36.7594, 5) centre (36.7594, 17) ccw
  arc A10 (25.8677, 11.963) -> (-25.8677, 11.963) centre (0, 0) ccw
  arc A11 (-36.7594, 5) -> (-25.8677, 11.963) centre (-36.7594, 17) ccw
  line L6 (-36.7594, 5) -> (-80, 5)
  line L7 (-80, 5) -> (-80, 3.5)
  line L8 (-80, 3.5) -> (-28.2843, 3.5)
  arc A12 (-28.2843, 3.5) -> (-28.2843, -3.5) centre (0, 0) ccw
  line L9 (-28.2843, -3.5) -> (-80, -3.5)
  line L10 (-80, -3.5) -> (-80, -5)
  line L11 (-80, -5) -> (-36.7594, -5)
  arc A13 (-25.8677, -11.963) -> (-36.7594, -5) centre (-36.7594, -17) ccw
  arc A14 (-25.8677, -11.963) -> (25.8677, -11.963) centre (0, 0) ccw
  circle A15 centre (0, 0) radius 17.5 construction
  line L12 (0, 0) -> (-26.7302, 13.6197) construction
  line L13 (0, 0) -> (-25.9808, -15) construction
  line L14 (-12.6727, 12.0687) -> (-25.1849, 17.3092) construction
  arc A16 (-25.1849, 17.3092) -> (-28.8068, 10.201) centre (-26.7302, 13.6197) ccw construction
  line L15 (-28.8068, 10.201) -> (-17.2126, 3.1586)
  line L16 (0, 0) -> (-17.5, 0) construction
  line L17 (-17.0237, -4.0551) -> (-28.2334, -11.6946)
  arc A17 (-28.2334, -11.6946) -> (-24.2445, -18.6035) centre (-25.9808, -15) ccw construction
  line L18 (-24.2445, -18.6035) -> (-12.0237, -12.7154) construction
  circle A18 centre (0, 0) radius 28.5
  line L19 (17.0237, 4.0551) -> (28.2334, 11.6946)
  line L20 (28.8068, -10.201) -> (17.2126, -3.1586)
  circle A19 centre (-25, 0) radius 3
  circle A20 centre (25, 0) radius 3
  dimension "d23" = 35
  dimension "d24" = 30
  dimension "d25" = 4
  dimension "d26" = 10
  dimension "d27" = 27
  dimension "d28" = 30
  dimension "d29" = 57
  dimension "d31" = 360
  dimension "d32" = 6
  constraint coincident A4.centre A8.centre
  constraint coincident A15 L14.start
  constraint tangent L14 A16
  constraint coincident A15 L15.end
  constraint tangent A16 L15
  constraint coincident L12.end A16.centre
  constraint symmetric L12 L14.start L15.end
  constraint coincident A15 L16.end
  constraint horizontal L16
  constraint coincident A15 L17.start
  constraint tangent L17 A17
  constraint coincident A15 L18.end
  constraint tangent A17 L18
  constraint coincident L13.end A17.centre
  constraint equal L12 L13
  constraint equal A16 A17
  constraint equal L15 L17
  constraint equal L17 L18
  constraint concentric A3 A19
  constraint concentric A0 A20
  constraint equal A19 A20
  measures "d23" diameter of A15
  measures "d24" distance of A4.centre L12.end
  measures "d25" radius of A16
  measures "d26" distance of L14.start L15.end
  measures "d27" angle of L12 L16
  measures "d28" angle of L13 L16
  measures "d29" diameter of A18
  measures "d32" diameter of A19
extrude "拉伸4" add sketch "草图3" along normal blind 8.4 contours A4 A8 A18 L19 L20 | A4 A12 L15 L17 A18
fillet "圆角2" radius 1 7 edges at (26.4921, 10.5079, 8.2) (-27.0058, 9.107, 8.2) (19.215, 5.5485, 8.2) (19.479, -4.5352, 8.2) (-26.4921, -10.5079, 8.2) (-19.215, -5.5485, 8.2) (27.0058, -9.107, 8.2)
extrude "拉伸5" cut sketch "草图1" against normal blind 5 from surface at 15 contours A9 | A10 | A11 | A12 | A13 | A14 | A15 | A16
sketch "草图4" plane through (80, 0, 0) normal (1, 0, 0) x (0, 1, 0)
  line L0 (5, 4) -> (3.5, 4)
  line L1 (3.5, 4) -> (3.5, 15)
  line L2 (3.5, 15) -> (-3.5, 15)
  line L3 (-3.5, 15) -> (-3.5, 4)
  line L4 (-3.5, 4) -> (-5, 4)
  line L5 (-5, 4) -> (-5, 0)
  line L6 (-5, 0) -> (5, 0)
  line L7 (5, 0) -> (5, 4)
  line L8 (-5, 0) -> (5, 0)
  line L9 (5, 0) -> (5, 20)
  line L10 (5, 20) -> (-5, 20)
  line L11 (-5, 20) -> (-5, 0)
  dimension "d41" = 20
  constraint horizontal L8
  constraint vertical L9
  constraint horizontal L10
  constraint vertical L11
  constraint coincident L5.end L6.start
  constraint coincident L6.end L7.start
  measures "d41" distance of L5.end L10.end
extrude "拉伸6" [suppressed]
mirror "镜像1" [suppressed]

design "M3铝柱 70mm"
part number: 2026-08-11-12-15-26-953
Autodesk Fusion 360 part; units mm, degrees
sketch "草图1" plane through (0, 0, 0) normal (0, 1, 0) x (1, 0, 0)
  circle A0 centre (0, 0) radius 1.5
  circle A1 centre (0, 0) radius 3
  dimension "d1" = 3
  dimension "d2" = 6
  constraint coincident A0.centre A1.centre
  constraint concentric A0 A1
  measures "d1" diameter of A0
  measures "d2" diameter of A1
extrude "拉伸1" add sketch "草图1" along normal mid plane 70 makes body 1
pattern_linear "R-阵列1" count 2 spacing 30 along (1, 0, 0) of bodies 1 makes body 2

design "夹爪连杆底座"
part number: 2026-07-21-18-51-26-851
Autodesk Fusion 360 part; units mm, degrees
sketch "草图1" plane through (0, 0, 0) normal (0, 0, 1) x (1, 0, 0)
  circle A0 centre (0, 0) radius 17.5
  circle A1 centre (0, 0) radius 13.5 construction
  line L0 (0, 0) -> (0, 17.5) construction
  circle A2 centre (0, 13.5) radius 1.6
  circle A3 centre (-11.6913, 6.75) radius 1.6
  circle A4 centre (-11.6913, -6.75) radius 1.6
  circle A5 centre (0, -13.5) radius 1.6
  circle A6 centre (11.6913, -6.75) radius 1.6
  circle A7 centre (11.6913, 6.75) radius 1.6
  dimension "d1" = 27
  dimension "d2" = 35
  dimension "d3" = 3.2
  dimension "d5" = 360
  constraint coincident A0.centre A1.centre
  constraint coincident A0 L0.end
  constraint vertical L0
  constraint coincident A1 A2.centre
  constraint coincident L0 A2.centre
  measures "d1" diameter of A1
  measures "d2" diameter of A0
  measures "d3" diameter of A2
extrude "拉伸1" add sketch "草图1" along normal blind 7 makes body 1
sketch "草图2" plane through (0, 0, 7) normal (0, 0, 1) x (-1, 0, 0)
  circle A0 centre (-11.6913, 6.75) radius 1.6
  circle A1 centre (0, -13.5) radius 1.6
  circle A2 centre (11.6913, 6.75) radius 1.6
  circle A3 centre (11.6913, -6.75) radius 1.6
  circle A4 centre (-11.6913, -6.75) radius 1.6
  circle A5 centre (0, 13.5) radius 1.6
  circle A6 centre (0, 0) radius 17.5
  line L0 (0, 0) -> (0, -17.5) construction
  line L1 (0, 0) -> (30, 0) construction
  circle A7 centre (30, 0) radius 1.25
  line L2 (16.7705, -5) -> (30.2981, -3.9889)
  arc A8 (30.2981, -3.9889) -> (30.2981, 3.9889) centre (30, 0) ccw
  line L3 (30.2981, 3.9889) -> (16.7705, 5)
  line L4 (-16.7705, -5) -> (-30.2981, -3.9889)
  arc A9 (-30.2981, 3.9889) -> (-30.2981, -3.9889) centre (-30, 0) ccw
  line L5 (-30.2981, 3.9889) -> (-16.7705, 5)
  circle A10 centre (-30, 0) radius 1.25
  circle A11 centre (30, 0) radius 2.5
  circle A12 centre (-30, 0) radius 2.5
  dimension "d8" = 2.5
  dimension "d9" = 60
  dimension "d10" = 10
  dimension "d11" = 4
  dimension "d15" = 5
  constraint coincident A6.centre L0.start
  constraint coincident A6 L0.end
  constraint vertical L0
  constraint perpendicular L0 L1
  constraint coincident L1.end A7.centre
  constraint coincident A6 L2.start
  constraint tangent L2 A8
  constraint coincident A6 L3.end
  constraint tangent A8 L3
  constraint coincident L1 A7.centre
  constraint symmetric L0 A7 A10
  constraint symmetric L0 L2.start L4.start
  constraint symmetric L0 L2.end L4.end
  constraint symmetric L0 A8.end A9.start
  constraint symmetric L0 A8 A9
  constraint symmetric L0 L3.end L5.end
  constraint symmetric L1 L2.start L3.end
  constraint concentric A7 A11
  constraint concentric A9 A12
  constraint equal A11 A12
  measures "d8" diameter of A7
  measures "d9" distance of L1.end A9.centre
  measures "d10" distance of L2.start L3.end
  measures "d11" radius of A8
  measures "d15" diameter of A11
extrude "拉伸2" add sketch "草图2" along normal blind 5 contours A6 | A6 L2 A8 L3 | A6 L4 A9 L5 | A11 | A12 bodies 1
extrude "拉伸6" add sketch "草图2" along normal blind 1 from surface at 5 separate body contours A11 | A12 makes body 2 at (27.5124, 0.2489, 12.3333) makes body 3 at (-32.4876, 0.2489, 12.3333)
fillet "圆角1" radius 3 4 edges at (-16.7705, -5, 9.5) (16.7705, -5, 9.5) (16.7705, 5, 9.5) (-16.7705, 5, 9.5) on bodies 1
sketch "草图3" plane through (0, 0, 12) normal (0, 0, 1) x (-1, 0, 0)
  arc A0 (-16.1674, -6.698) -> (16.1674, -6.698) centre (0, 0) ccw
  arc A1 (18.7154, -4.8546) -> (16.1674, -6.698) centre (18.939, -7.8463) ccw
  line L0 (18.7154, -4.8546) -> (30.2981, -3.9889)
  arc A2 (30.2981, -3.9889) -> (30.2981, 3.9889) centre (30, 0) ccw
  line L1 (30.2981, 3.9889) -> (18.7154, 4.8546)
  arc A3 (16.1674, 6.698) -> (18.7154, 4.8546) centre (18.939, 7.8463) ccw
  arc A4 (16.1674, 6.698) -> (-16.1674, 6.698) centre (0, 0) ccw
  arc A5 (-18.7154, 4.8546) -> (-16.1674, 6.698) centre (-18.939, 7.8463) ccw
  line L2 (-18.7154, 4.8546) -> (-30.2981, 3.9889)
  arc A6 (-30.2981, 3.9889) -> (-30.2981, -3.9889) centre (-30, 0) ccw
  line L3 (-30.2981, -3.9889) -> (-18.7154, -4.8546)
  arc A7 (-16.1674, -6.698) -> (-18.7154, -4.8546) centre (-18.939, -7.8463) ccw
  circle A8 centre (0, 13.5) radius 1.6
  circle A9 centre (-11.6913, -6.75) radius 1.6
  circle A10 centre (0, -13.5) radius 1.6
  circle A11 centre (11.6913, -6.75) radius 1.6
  circle A12 centre (11.6913, 6.75) radius 1.6
  circle A13 centre (-11.6913, 6.75) radius 1.6
  circle A14 centre (11.6913, -6.75) radius 3
  circle A15 centre (11.6913, 6.75) radius 3
  circle A16 centre (0, 13.5) radius 3
  circle A17 centre (-11.6913, 6.75) radius 3
  circle A18 centre (-11.6913, -6.75) radius 3
  circle A19 centre (0, -13.5) radius 3
  circle A20 centre (30, 0) radius 1.25
  circle A21 centre (-30, 0) radius 1.25
  dimension "d21" = 6
  dimension "d23" = 360
  constraint concentric A11 A14
  measures "d21" diameter of A14
extrude "拉伸4" cut sketch "草图3" against normal blind 3.5 contours A14 | A15 | A16 | A17 | A18 | A19 bodies 1